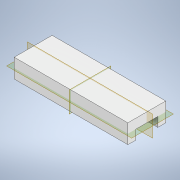
# Autodesk Inventor part: forkmount
Saved by Autodesk Inventor 2022 (Build 260153000, 153)
## iProperties
Created: 2022-10-23
Part Number: forkmount
Material: ABS プラスチック
Document SubType Name: Modeling
Designer: Yazawa
Density: 1.06 g/cm^3
Appearance: 滑らか - 白
Mass: 9.02853 g
Surface Area: 44.8756 cm^2
Volume: 8.51748 cm^3
Author: Yazawa
Autodesk Inventor part; units mm, degrees
ref_plane "YZ Plane" through (0, 0, 0) normal (1, 0, 0) x (0, 1, 0)
ref_plane "XZ Plane" through (0, 0, 0) normal (0, 1, 0) x (-1, 0, 0)
ref_plane "XY Plane" through (0, 0, 0) normal (0, 0, 1) x (1, 0, 0)
sketch "スケッチ1" plane through (0, 0, 0) normal (0, 1, 0) x (-1, 0, 0)
  line L0 (30, -10) -> (-30, -10)
  line L1 (-30, -10) -> (-30, 10)
  line L2 (-30, 10) -> (30, 10)
  line L3 (30, 10) -> (30, -10)
  line L4 (30, -10) -> (-30, 10) construction
  line L5 (30, 10) -> (-30, -10) construction
  point P0 (0, 0)
  point P1 (0, 0)
  dimension "d0" = 60
  dimension "d1" = 20
  constraints: 12 end point, 2 parallel, 1 coincident, 1 horizontal, 1 midpoint, 1 perpendicular
  measures "d0" distance of L0.start L0.end
  measures "d1" distance of L2.end L0.start
extrude "押し出し1" add sketch "スケッチ1" along normal blind 10
sketch "スケッチ3" plane through (0, 0, 0) normal (0, -1, 0) x (1, 0, 0)
  line L0 (30, 5.8) -> (-30, 5.8)
  line L1 (-30, 5.8) -> (-30, -5.8)
  line L2 (-30, -5.8) -> (30, -5.8)
  line L3 (30, -5.8) -> (30, 5.8)
  line L4 (30, 10) -> (30, -10) projected
  line L5 (-30, -10) -> (-30, 10) projected
  line L6 (30, 5.8) -> (-30, -5.8) construction
  point P0 (0, 0)
  point P1 (0, 0)
  dimension "d12" = 11.6
  constraints: 10 end point, 2 collinear, 2 parallel, 1 coincident, 1 horizontal, 1 midpoint, 1 perpendicular
  measures "d12" distance of L2.end L0.start
extrude "押し出し2" cut sketch "スケッチ3" against normal blind 5
sketch "スケッチ4" plane through (0, 5, 0) normal (0, -1, 0) x (1, 0, 0)
  line L0 (-25, 0) -> (25, 0) construction
  point P0 (0, 0)
  point P1 (0, 0)
  dimension "d15" = 50
  constraints: 2 end point, 1 coincident, 1 horizontal, 1 horizontal alignment, 1 midpoint
  measures "d15" distance of L0.start L0.end
hole "穴2" at (-25, 5, 0) at (25, 5, 0) direction (0, 1, 0) diameter 2 depth 0.2 tip angle 118
ref_plane "作業平面1" through (0, 0, 10) normal (-1, 0, 0) x (0, 0, 1)
ref_plane "作業平面2" through (-30, 0, 0) normal (0, 0, 1) x (1, 0, 0)
ref_plane "作業平面3" through (0, 5, 0) normal (0, -1, 0) x (1, 0, 0)
